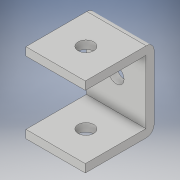
# Autodesk Inventor part: RobotArm CylinderPart2
Saved by Autodesk Inventor 2018 (Build 220112000, 112)
## iProperties
Created: 2018-01-20
Part Number: RobotArm CylinderPart2
Material: Generic
Document SubType Name: Modeling
Designer: lopez.xavier
Density: 1 g/cm^3
Appearance: Default
Author: lopez.xavier
Autodesk Inventor part; units mm, degrees
ref_plane "YZ Plane" through (0, 0, 0) normal (1, 0, 0) x (0, 1, 0)
ref_plane "XZ Plane" through (0, 0, 0) normal (0, 1, 0) x (-1, 0, 0)
ref_plane "XY Plane" through (0, 0, 0) normal (0, 0, 1) x (1, 0, 0)
sketch "Sketch1" plane through (0, 0, 0) normal (0, 0, 1) x (1, 0, 0)
  line L0 (0, 0) -> (24.13, 0)
  line L1 (24.13, 0) -> (24.13, -32.385)
  line L2 (24.13, -32.385) -> (0, -32.385)
  line L3 (0, -32.385) -> (0, 0)
  dimension "d0" = 24.13
  dimension "d1" = 32.385
  constraints: 8 end point, 2 parallel, 1 horizontal, 1 perpendicular
  measures "d0" distance of L1.end L2.end
  measures "d1" distance of L0.end L1.end
extrude "Extrusion1" add sketch "Sketch1" along normal blind 27.94
sketch "Sketch2" plane through (24.13, -32.385, 0) normal (1, 0, 0) x (0, 0, -1)
  line L0 (-27.94, 29.083) -> (-3.302, 29.083)
  line L1 (-3.302, 29.083) -> (-3.302, 3.302)
  line L2 (-3.302, 3.302) -> (-27.94, 3.302)
  line L3 (-27.94, 3.302) -> (-27.94, 29.083)
  line L4 (-27.94, 0) -> (-27.94, 32.385) projected
  line L5 (0, 0) -> (-27.94, 0) projected
  line L6 (0, 32.385) -> (0, 0) projected
  line L7 (0, 32.385) -> (-27.94, 32.385) projected
  dimension "d4" = 0
  dimension "d5" = 3.302
  dimension "d6" = 3.302
  dimension "d7" = 3.302
  constraints: 8 end point, 2 parallel, 1 horizontal, 1 perpendicular
  measures "d4" distance between parallel lines of L4 L3
  measures "d5" distance between parallel lines of L5 L2
  measures "d6" distance between parallel lines of L6 L1
  measures "d7" distance between parallel lines of L7 L0
extrude "Extrusion2" cut sketch "Sketch2" against normal blind 34.925 contours L0 L1 L2 L3
sketch "Sketch3" plane through (24.13, -29.083, 3.302) normal (0, 0, 1) x (1, 0, 0)
  line L0 (-24.13, 0) -> (-24.13, 25.781) projected
  line L1 (0, 0) -> (-24.13, 0) projected
  line L2 (0, 25.781) -> (0, 0) projected
  line L3 (0, 25.781) -> (-24.13, 25.781) projected
  line L4 (-24.13, 25.781) -> (0, 25.781) projected
  line L5 (-12.065, 25.781) -> (-12.065, 0)
  line L6 (0, 0) -> (-24.13, 0) projected
  line L7 (-24.13, 0) -> (-24.13, 25.781) projected
  line L8 (-24.13, 12.8905) -> (0, 12.8905)
  circle A0 centre (-12.065, 12.8905) radius 3.175
  point P0 (-24.13, 29.083)
  dimension "d10" = 6.35
  constraints: 5 midpoint, 4 end point, 1 centre point
  measures "d10" diameter of A0
extrude "Extrusion3" cut sketch "Sketch3" against normal blind 34.925 contours A0 L5 L8 | L8 L5 A0 | L5 L8 A0 | L5 A0 L8
fillet "Fillet1" radius 3.175 2 edges at (12.065, 0, 0) (12.065, -32.385, 0)
sketch "Sketch4" plane through (0, 0, 27.94) normal (0, 1, 0) x (1, 0, 0)
  circle A0 centre (12.065, 12.319) radius 3.175
  line L0 (24.13, 24.765) -> (24.13, 0) projected
  line L1 (24.13, 0) -> (0, 0) projected
  point P0 (0, 27.94)
  dimension "d14" = 6.35
  dimension "d15" = 12.065
  dimension "d16" = 12.319
  constraints: 1 centre point
  measures "d14" diameter of A0
  measures "d15" distance from line of L0 A0.centre
  measures "d16" distance from line of L1 A0.centre
extrude "Extrusion4" cut sketch "Sketch4" against normal blind 34.925
body "Solid1"
